spessorialtifrigobosch (Autodesk Fusion 360 design; units mm, degrees)
Autodesk Fusion 360 part; units mm, degrees
sketch "Sketch1" plane through (0, 0, 0) normal (0, 0, 1) x (1, 0, 0)
  line L0 (21, -22.5) -> (-21, -22.5)
  line L1 (-21, -22.5) -> (-21, 22.5)
  line L2 (-21, 22.5) -> (21, 22.5)
  line L3 (21, 22.5) -> (21, -22.5)
  line L4 (21, -22.5) -> (-21, 22.5) construction
  line L5 (-21, -22.5) -> (21, 22.5) construction
  line L6 (0, 22.5) -> (0, -22.5)
  line L7 (-21, 0) -> (21, 0)
  line L8 (17.6, 19) -> (17.6, 7)
  line L9 (17.6, -7.9) -> (17.6, -19.9)
  line L10 (11.8, 19) -> (11.8, 7)
  line L11 (11.8, -7.9) -> (11.8, -19.9)
  line L12 (-11.8, 19) -> (-11.8, 7)
  line L13 (-11.8, -7.9) -> (-11.8, -19.9)
  line L14 (-17.6, 19) -> (-17.6, 7)
  line L15 (-17.6, -7.9) -> (-17.6, -19.9)
  line L16 (-17.7333, 19) -> (-11.8, 19)
  line L17 (11.8, 19) -> (17.7333, 19)
  line L18 (-17.6, 7) -> (-11.8, 7)
  line L19 (11.8, 7) -> (17.6, 7)
  line L20 (-17.6, -7.9) -> (-11.8, -7.9)
  line L21 (11.8, -7.9) -> (17.6, -7.9)
  line L22 (-17.6, -19.9) -> (-11.8, -19.9)
  line L23 (11.8, -19.9) -> (17.6, -19.9)
  dimension "d1" = 42
  dimension "d2" = 45
  dimension "d5" = 3.5
  dimension "d6" = 15.5
  dimension "d7" = 30.4
  dimension "d8" = 42.4
  constraint horizontal L0
  constraint perpendicular L0 L1
  constraint parallel L0 L2
  constraint parallel L1 L3
  constraint coincident L4 origin
  constraint coincident L5 origin
  constraint midpoint L2 L6.start
  constraint midpoint L0 L6.end
  constraint midpoint L1 L7.start
  constraint midpoint L3 L7.end
  constraint perpendicular L0 L14
  constraint perpendicular L3 L16
  constraint perpendicular L3 L18
  constraint perpendicular L3 L20
  constraint perpendicular L3 L22
  constraint coincident L14.start L16
  constraint coincident L10.start L16
  constraint coincident L8.start L16
  constraint coincident L8.end L18
  constraint collinear L8 L9
  constraint coincident L10.end L18
  constraint collinear L10 L11
  constraint collinear L12 L13
  constraint collinear L14 L15
  constraint coincident L4 L16.start
  constraint collinear L16 L17
  constraint collinear L18 L19
  constraint coincident L5 L17.end
  constraint coincident L11.start L20
  constraint coincident L9.start L20
  constraint coincident L9.end L22
  constraint coincident L11.end L22
  constraint collinear L20 L21
  constraint collinear L22 L23
  measures "d1" distance of L1.end L2.end
  measures "d2" distance of L0.end L1.end
  measures "d5" distance of L2 L16
  measures "d6" distance of L2 L18
  measures "d7" distance of L2 L20
  measures "d8" distance of L2 L22
extrude "Extrude1" add sketch "Sketch1" along normal blind 3
fillet "Fillet1" radius 2 4 edges at (-21, 22.5, 1.5) (21, 22.5, 1.5) (21, -22.5, 1.5) (-21, -22.5, 1.5)
fillet "Fillet2" radius 2 4 edges at (17.6, 7, 1.5) (11.8, 7, 1.5) (11.8, 19, 1.5) (17.6, 19, 1.5)
fillet "Fillet3" radius 2 4 edges at (-17.6, 19, 1.5) (-11.8, 19, 1.5) (-11.8, 7, 1.5) (-17.6, 7, 1.5)
fillet "Fillet4" radius 2 4 edges at (-11.8, -19.9, 1.5) (-17.6, -19.9, 1.5) (-17.6, -7.9, 1.5) (-11.8, -7.9, 1.5)
fillet "Fillet5" radius 2 4 edges at (11.8, -7.9, 1.5) (17.6, -7.9, 1.5) (11.8, -19.9, 1.5) (17.6, -19.9, 1.5)
